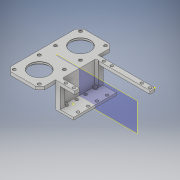
# Autodesk Inventor part: x_carriage_to_extruder
Saved by Autodesk Inventor 2019 (Build 230136000, 136)
## iProperties
Created: 2020-04-12
Part Number: x_carriage_to_extruder
Material: Generisch
Document SubType Name: Modeling
Designer: marc
Density: 1 g/cm^3
Appearance: Vorgabe
Author: marc
Autodesk Inventor part; units mm, degrees
ref_plane "YZ Plane" through (0, 0, 0) normal (1, 0, 0) x (0, 1, 0)
ref_plane "XZ Plane" through (0, 0, 0) normal (0, 1, 0) x (-1, 0, 0)
ref_plane "XY Plane" through (0, 0, 0) normal (0, 0, 1) x (1, 0, 0)
sketch "Skizze1" plane through (0, 0, 0) normal (0, 1, 0) x (-1, 0, 0)
  line L0 (0, 0) -> (70, 0)
  line L1 (70, 0) -> (70, 53)
  line L2 (0, 6) -> (0, 0)
  line L3 (70, 53) -> (0, 53)
  line L4 (0, 53) -> (0, 47)
  line L5 (0, 47) -> (64, 47)
  line L6 (64, 47) -> (64, 6)
  line L7 (64, 6) -> (0, 6)
  dimension "d4" = 53
  dimension "d5" = 6
  dimension "d6" = 6
  dimension "d7" = 70
  dimension "d8" = 6
  constraints: 16 end point, 4 perpendicular, 2 horizontal, 1 parallel, 1 vertical, 1 vertical alignment
  measures "d4" distance between parallel lines of L0 L3
  measures "d5" distance of L2.start L0.start
  measures "d6" distance between parallel lines of L1 L6
  measures "d7" distance of L0.start L0.end
  measures "d8" distance of L3.end L4.end
extrude "Extrusion1" add sketch "Skizze1" along normal blind 4
sketch "Skizze2" plane through (0, 4, 0) normal (0, 1, 0) x (1, 0, 0)
  point P0 (0, 0)
sketch "Skizze3" plane through (-70, 0, 53) normal (0, 0, 1) x (1, 0, 0)
  line L0 (70, 0) -> (0, 0) projected
  line L1 (25, 0) -> (50, 0)
  line L2 (50, 0) -> (50, 1.8)
  line L3 (50, 1.8) -> (25, 1.8)
  line L4 (25, 1.8) -> (25, 0)
  line L5 (70, 0) -> (70, 4) projected
  dimension "d11" = 1.8
  dimension "d12" = 25
  dimension "d13" = 20
  constraints: 8 end point, 2 parallel, 1 horizontal, 1 perpendicular, 1 point on line
  measures "d11" distance of L1.end L2.end
  measures "d12" distance of L2.end L3.end
  measures "d13" distance between parallel lines of L5 L2
extrude "Extrusion2" cut sketch "Skizze3" against normal up to surface (6 mm away)
sketch "Skizze4" plane through (0, 4, 0) normal (0, 1, 0) x (1, 0, 0)
  line L0 (0, -53) -> (0, -47) projected
  line L1 (-70, -53) -> (0, -53) projected
  line L2 (-64, -6) -> (0, -6) projected
  point P0 (0, 0)
  point P1 (-3, -50)
  point P2 (-3, -3)
  point P3 (-60, -50)
  point P4 (-60, -3)
  point P5 (-50, -3)
  point P6 (-50, -50)
  point P7 (-13, -50)
  point P8 (-13, -3)
  dimension "d20" = 3
  dimension "d21" = 3
  dimension "d22" = 6
  dimension "d23" = 3
  dimension "d24" = 10
  dimension "d25" = 37
  dimension "d26" = 10
  constraints: 6 horizontal alignment, 4 vertical alignment
  measures "d20" distance from line of L0 point (-3, -50)
  measures "d21" distance from line of L1 point (-3, -50)
  measures "d22" distance of L0.start L0.end
  measures "d23" distance from line of L2 point (-3, -3)
  measures "d24" distance of point (-3, -50) point (-13, -50)
  measures "d25" distance of point (-50, -50) point (-13, -50)
  measures "d26" distance of point (-50, -50) point (-60, -50)
hole "Bohrung1" at (-60, 4, 50) at (-50, 4, 50) at (-13, 4, 50) at (-3, 4, 50) at (-3, 4, 3) at (-13, 4, 3) at (-50, 4, 3) at (-60, 4, 3) direction (0, -1, 0) diameter 3.6 end through all clearance for "Flachkopfsenkschraube DIN EN ISO 2009" size "M3" standard "DIN"
chamfer "Fase2" distance 1 angle 45 2 edges at (0, 4, 50) (0, 4, 3)
sketch "Skizze6" plane through (0, 0, 0) normal (0, -1, 0) x (1, 0, 0)
  line L0 (-64, 6) -> (-1, 6) projected
  line L1 (-64, 6) -> (-64, 0)
  line L2 (-1, 0) -> (-70, 0) projected
  line L3 (-1, 47) -> (-64, 47) projected
  line L4 (-64, 47) -> (-64, 53)
  line L5 (-70, 53) -> (-1, 53) projected
  line L6 (-64, 47) -> (-64, 6) projected
  line L7 (-70, 0) -> (-70, 53) projected
  point P0 (0, 0)
  constraints: 4 end point, 3 point on line, 1 vertical
extrude "Extrusion3" add sketch "Skizze6" along normal blind 25
sketch "Skizze8" plane through (0, -25, 0) normal (0, -1, 0) x (1, 0, 0)
  line L0 (-70, 0) -> (-70, 53) projected
  line L1 (-70, 53) -> (-54, 53)
  line L2 (-54, 53) -> (-54, 0)
  line L3 (-54, 0) -> (-70, 0)
  line L4 (-70, 0) -> (-70, 53)
  point P0 (0, 0)
  dimension "d40" = 16
  constraints: 8 end point, 2 parallel, 1 horizontal, 1 perpendicular, 1 point on line
  measures "d40" distance of L2.end L3.end
extrude "Extrusion4" add sketch "Skizze8" along normal blind 3
move faces "Verschieben1" translate (6.5, 0, 0) faces at (-54, -27, 17.6667)
sketch "Skizze9" plane through (0, -28, 0) normal (0, -1, 0) x (1, 0, 0)
  line L0 (-70, 53) -> (-70, 0) projected
  line L1 (-47.5, 53) -> (-70, 53) projected
  point P0 (0, 0)
  point P1 (-64.6, 8.5)
  point P2 (-64.6, 21)
  point P3 (-64.6, 32)
  point P4 (-64.6, 44.5)
  point P5 (-50.6, 21)
  point P6 (-50.6, 8.5)
  point P7 (-50.6, 32)
  point P8 (-50.6, 44.5)
  dimension "d43" = 5.4
  dimension "d44" = 12.5
  dimension "d45" = 14
  dimension "d49" = 12.5
  dimension "d50" = 11
  dimension "d51" = 53
  dimension "d52" = 36
  dimension "d53" = 8.5
  constraints: 6 vertical alignment, 4 horizontal alignment
  measures "d43" distance from line of L0 point (-64.6, 21)
  measures "d44" distance of point (-64.6, 8.5) point (-64.6, 21)
  measures "d45" distance of point (-50.6, 21) point (-64.6, 21)
  measures "d49" distance of point (-64.6, 44.5) point (-64.6, 32)
  measures "d50" distance of point (-64.6, 21) point (-64.6, 32)
  measures "d51" distance of L0.start L0.end
  measures "d52" distance of point (-64.6, 8.5) point (-64.6, 44.5)
  measures "d53" distance from line of L1 point (-64.6, 44.5)
hole "Bohrung2" at (-50.6, -28, 8.5) at (-50.6, -28, 21) at (-64.6, -28, 8.5) at (-64.6, -28, 21) at (-50.6, -28, 32) at (-50.6, -28, 44.5) at (-64.6, -28, 44.5) at (-64.6, -28, 32) direction (0, 1, 0) diameter 3.6 end through all clearance for "Flachkopfsenkschraube DIN EN ISO 2009" size "M3" standard "DIN"
sketch "Skizze11" plane through (0, 4, 0) normal (0, 1, 0) x (1, 0, 0)
  arc A0 (-64, -42.8029) -> (-64, -46.1971) centre (-64.6, -44.5) ccw projected
  arc A1 (-64, -19.3029) -> (-64, -22.6971) centre (-64.6, -21) ccw projected
  arc A2 (-64, -6.8029) -> (-64, -10.1971) centre (-64.6, -8.5) ccw projected
  line L0 (-67.45, -42.8546) -> (-64.6, -41.2091)
  line L1 (-64.6, -41.2091) -> (-61.75, -42.8546)
  line L2 (-61.75, -42.8546) -> (-61.75, -46.1454)
  line L3 (-61.75, -46.1454) -> (-64.6, -47.7909)
  line L4 (-64.6, -47.7909) -> (-67.45, -46.1454)
  line L5 (-67.45, -46.1454) -> (-67.45, -42.8546)
  line L6 (-64.6, -11.7909) -> (-67.45, -10.1454)
  line L7 (-67.45, -10.1454) -> (-67.45, -6.8546)
  line L8 (-67.45, -6.8546) -> (-64.6, -5.2091)
  line L9 (-64.6, -5.2091) -> (-61.75, -6.8546)
  line L10 (-61.75, -6.8546) -> (-61.75, -10.1454)
  line L11 (-61.75, -10.1454) -> (-64.6, -11.7909)
  line L12 (-64, -42.8029) -> (-64, -22.6971) projected
  line L13 (-64.6, -24.2909) -> (-67.45, -22.6454)
  line L14 (-67.45, -22.6454) -> (-67.45, -19.3546)
  line L15 (-67.45, -19.3546) -> (-64.6, -17.7091)
  line L16 (-64.6, -17.7091) -> (-61.75, -19.3546)
  line L17 (-61.75, -19.3546) -> (-61.75, -22.6454)
  line L18 (-61.75, -22.6454) -> (-64.6, -24.2909)
  line L19 (-47.5, 0) -> (-47.5, -53) projected
  arc A3 (-64, -30.3029) -> (-64, -33.6971) centre (-64.6, -32) ccw projected
  line L20 (-64.6, -35.2909) -> (-67.45, -33.6454)
  line L21 (-67.45, -33.6454) -> (-67.45, -30.3546)
  line L22 (-67.45, -30.3546) -> (-64.6, -28.7091)
  line L23 (-64.6, -28.7091) -> (-61.75, -30.3546)
  line L24 (-61.75, -30.3546) -> (-61.75, -33.6454)
  line L25 (-61.75, -33.6454) -> (-64.6, -35.2909)
  point P0 (0, 0)
  dimension "d62" = 5.7
  dimension "d64" = 5.7
  constraints: 48 end point, 6 coincident, 4 vertical alignment, 2 parallel, 52 other
  measures "d62" distance between parallel lines of L3 L0
  measures "d64" distance between parallel lines of L24 L21
extrude "Extrusion5" cut sketch "Skizze11" against normal blind 27 contours L0 L1 L2 L3 L4 L5 | L6 L7 L8 L9 L10 L11 | L12 L23 L24 L25 | L12 L25 L20 L21 L22 L23 A3 | L13 L14 L15 L16 L17 L18
sketch "Skizze12" plane through (0, 4, 0) normal (0, 1, 0) x (1, 0, 0)
  line L0 (-61.75, -6.8546) -> (-61.75, -10.1454) projected
  line L1 (-67.45, -42.8546) -> (-64.6, -41.2091) projected
  line L2 (-61.75, -10.1454) -> (-67.45, -10.1454)
  line L3 (-67.45, -10.1454) -> (-67.45, -42.8546)
  line L4 (-67.45, -42.8546) -> (-61.75, -42.8546)
  line L5 (-61.75, -42.8546) -> (-61.75, -10.1454)
  point P0 (0, 0)
  constraints: 8 end point, 2 parallel, 1 horizontal, 1 perpendicular
extrude "Extrusion6" cut sketch "Skizze12" against normal up to surface (29 mm away)
chamfer "Fase3" distance 1.7 angle 45 2 edges at (-20, 1.8, 50) (-45, 1.8, 50)
fillet "Rundung1" radius 2 2 edges at (-20, 0, 50) (-45, 0, 50)
chamfer "Fase4" [suppressed]
sketch "Skizze13" plane through (-64.6, -23, 47.7909) normal (0.5, 0, -0.8660254) x (-0.8660254, 0, -0.5)
  point P0 (-32.0498, 23)
sketch "Skizze15" plane through (0, 0, 0) normal (0, 0, -1) x (-1, 0, 0)
  line L0 (68.3, -28) -> (70, -26.3) projected
  line L1 (70, -26.3) -> (91.2132, -5.0868)
  line L2 (70, -26.3) -> (100, -26.3) construction
  line L3 (91.2132, -5.0868) -> (88.3848, -2.2584)
  line L4 (88.3848, -2.2584) -> (70, -20.6431)
  line L5 (70, -28) -> (70, 4) projected
  point P0 (0, 0)
  point P1 (70, 2.3)
  dimension "d80" = 30
  dimension "d81" = 45
  dimension "d82" = 4
  constraints: 8 end point, 2 perpendicular, 1 collinear, 1 equal length, 1 horizontal, 1 point on line
  measures "d80" distance of L0.end L1.end
  measures "d81" angle of L2 L1
  measures "d82" distance of L1.end L3.end
extrude "Extrusion8" [suppressed]
sketch "Skizze16" plane through (-68.3, -28, 53) normal (-0.7071068, -0.7071068, 0) x (-0.7071068, 0.7071068, 0)
  line L0 (0, 0) -> (2.4042, 0) projected
  line L1 (32.4042, 53) -> (32.4042, 0) projected
  point P0 (-28.4964, 53)
  point P1 (27.0042, 8.5)
  point P2 (13.0042, 8.5)
  point P3 (27.0042, 21)
  point P4 (13.0042, 21)
  point P5 (27.0042, 32)
  point P6 (13.0042, 32)
  point P7 (27.0042, 44.5)
  point P8 (13.0042, 44.5)
  dimension "d85" = 8.5
  dimension "d86" = 36
  dimension "d87" = 11
  dimension "d88" = 12.5
  dimension "d89" = 14
  dimension "d90" = 5.4
  constraints: 6 vertical alignment, 4 horizontal alignment
  measures "d85" distance from line of L0 point (27.004, 8.5)
  measures "d86" distance of point (27.004, 44.5) point (27.004, 8.5)
  measures "d87" distance of point (27.004, 32) point (27.004, 21)
  measures "d88" distance of point (27.004, 44.5) point (27.004, 32)
  measures "d89" distance of point (27.004, 21) point (13.004, 21)
  measures "d90" distance from line of L1 point (27.004, 21)
hole "Bohrung3" [suppressed]
sketch "Skizze17" plane through (0, 0, 53) normal (0, 0, 1) x (1, 0, 0)
  line L0 (-46.2285, 0) -> (0, 0)
  line L1 (0, 0) -> (0, 4)
  line L2 (0, 4) -> (-46.2285, 4)
  line L3 (-46.2285, 4) -> (-46.2285, 0)
  line L4 (-64, 0) -> (-45.6245, 0) projected
  point P0 (0, 0)
  point P1 (-1, 4)
  dimension "d98" = 46.2285
  constraints: 8 end point, 4 point on line, 2 parallel, 1 horizontal, 1 perpendicular
  measures "d98" distance of L1.end L2.end
extrude "Extrusion9" cut sketch "Skizze17" against normal up to surface (6 mm away)
fillet "Rundung2" [suppressed]
sketch "Skizze18" plane through (0, 0, 0) normal (0, 0, -1) x (-1, 0, 0)
  line L0 (70, -28) -> (70, 4) projected
  line L1 (70, -7.7) -> (94.7487, -32.4487)
  line L2 (70, 2.3) -> (105, 2.3) construction
  line L3 (94.7487, -32.4487) -> (91.9203, -35.2772)
  line L4 (91.9203, -35.2772) -> (70, -13.3569)
  line L5 (70, -28) -> (70, 4) projected
  point P0 (0, 0)
  point P1 (70, -26.3)
  dimension "d102" = 35
  dimension "d103" = 45
  dimension "d104" = 4
  dimension "d126" = 10
  constraints: 8 end point, 2 perpendicular, 2 point on line, 1 equal length, 1 horizontal
  measures "d102" distance of L1.start L1.end
  measures "d103" angle of L1 L2
  measures "d104" distance of L1.end L3.end
  measures "d126" distance of L2.start L1.start
extrude "Extrusion10" [suppressed]
sketch "Skizze19" plane through (-68.3, 4, 0) normal (-0.7071068, 0.7071068, 0) x (-0.7071068, -0.7071068, 0)
  line L0 (2.4042, 53) -> (0, 53) projected
  line L1 (0, 53) -> (0, 0) projected
  line L2 (9.4752, 0) -> (9.4752, 53) projected
  point P0 (-45.467, 0)
  point P1 (40.4752, 44.5)
  point P2 (40.4752, 32)
  point P3 (26.4752, 44.5)
  point P4 (26.4752, 32)
  point P5 (26.4752, 21)
  point P6 (26.4752, 8.5)
  point P7 (40.4752, 21)
  point P8 (40.4752, 8.5)
  point P9 (32.4042, 53)
  dimension "d107" = 8.5
  dimension "d108" = 36
  dimension "d109" = 12.5
  dimension "d110" = 11
  dimension "d112" = 14
  dimension "d128" = 17
  constraints: 6 vertical alignment, 4 horizontal alignment
  measures "d107" distance from line of L0 point (40.475, 44.5)
  measures "d108" distance of point (26.475, 8.5) point (26.475, 44.5)
  measures "d109" distance of point (26.475, 44.5) point (26.475, 32)
  measures "d110" distance of point (26.475, 32) point (26.475, 21)
  measures "d112" distance of point (40.475, 32) point (26.475, 32)
  measures "d128" distance from line of L2 point (26.475, 44.5)
hole "Bohrung4" [suppressed]
sketch "Skizze20" plane through (0, 0, 0) normal (0, 0, -1) x (-1, 0, 0)
  line L0 (70, -13.3569) -> (91.9203, -35.2772) projected
  line L1 (76.4716, -19.8284) -> (70, -19.8284)
  line L2 (70, -28) -> (70, 4) projected
  point P0 (0, 0)
  point P1 (70, -26.3)
  point P2 (70, 2.3)
  dimension "d120" = 90
  constraints: 2 end point, 2 point on line
  measures "d120" angle of L2 L1
extrude "Extrusion11" [suppressed]
ref_plane "Arbeitsebene1" through (0, 0, 26.5) normal (0, 0, -1) x (-1, 0, 0)
mirror "Spiegeln1" [suppressed]
pattern_linear "Rechteckige Anordnung1" [suppressed]
sketch "Skizze21" plane through (-70, 4, 0) normal (-1, 0, 0) x (0, 0, 1)
  line L0 (53, -32) -> (53, 0) projected
  line L1 (0, 0) -> (53, 0)
  line L2 (53, 0) -> (53, -4)
  line L3 (53, -4) -> (0, -4)
  line L4 (0, -4) -> (0, 0)
  point P0 (0, -4)
  dimension "d129" = 4
  constraints: 8 end point, 2 parallel, 1 coincident, 1 horizontal, 1 perpendicular, 1 point on line
  measures "d129" distance of L0.end L2.end
extrude "Extrusion12" add sketch "Skizze21" along normal blind 42
sketch "Skizze22" plane through (0, 4, 0) normal (0, 1, 0) x (1, 0, 0)
  line L0 (-134.4, -26.5) -> (22.4, -26.5) projected
  line L1 (-70, -53) -> (-70, 0) projected
  line L2 (-70, -53) -> (-70, 0) projected
  line L3 (-1, 0) -> (-112, 0) projected
  point P0 (0, 0)
  point P1 (-106.5, -16.5)
  point P2 (-75.5, -16.5)
  point P3 (-106.5, 14.5)
  point P4 (-75.5, 14.5)
  dimension "d132" = 10
  dimension "d133" = 31
  dimension "d134" = 5.5
  dimension "d135" = 16.5
  dimension "d138" = 31
  dimension "d139" = 31
  constraints: 2 horizontal alignment, 1 vertical alignment
  measures "d132" distance from line of L0 point (-106.5, -16.5)
  measures "d133" distance of point (-106.5, -16.5) point (-75.5, -16.5)
  measures "d134" distance from line of L1 point (-75.5, -16.5)
  measures "d135" distance from line of L3 point (-75.5, -16.5)
  measures "d138" distance of point (-106.5, -16.5) point (-106.5, 14.5)
  measures "d139" distance of point (-75.5, -16.5) point (-75.5, 14.5)
sketch "Skizze23" plane through (0, 0, 0) normal (0, 0, -1) x (-1, 0, 0)
  line L0 (1, 4) -> (112, 4) projected
  line L1 (112, 0) -> (70, 0)
  line L2 (70, 0) -> (70, 4)
  line L3 (70, 4) -> (112, 4)
  line L4 (112, 4) -> (112, 0)
  point P0 (0, 0)
  point P1 (75.5, 4)
  point P2 (106.5, 4)
  constraints: 8 end point, 2 parallel, 2 point on line, 1 coincident, 1 horizontal, 1 perpendicular
extrude "Extrusion13" add sketch "Skizze23" along normal blind 25.5
hole "Bohrung5" at (-106.5, 4, -14.5) at (-106.5, 4, 16.5) at (-75.5, 4, 16.5) at (-75.5, 4, -14.5) direction (0, -1, 0) diameter 3.4 end through all
sketch "Skizze24" plane through (0, 4, 0) normal (0, 1, 0) x (1, 0, 0)
  circle A0 centre (-106.5, -16.5) radius 1.7 projected
  point P0 (0, 0)
  point P1 (-91, -1)
  dimension "d147" = 15.5
  dimension "d148" = 15.5
  measures "d147" horizontal distance of A0.centre point (-91, -1)
  measures "d148" horizontal distance of A0.centre point (-91, -1)
hole "Bohrung6" at (-91, 4, 1) direction (0, -1, 0) diameter 24 end through all
chamfer "Fase5" distance 2 angle 45 1 edges at (-91, 0, -11)
move faces "Verschieben2" translate (0, 0, 6.5) faces at (-98, 1.3333, -25.5)
chamfer "Fase6" distance 5.25 angle 45 2 edges at (-70, 2, -19) (-112, 2, -19)
mirror "Spiegeln3" about plane through (0, 0, 26.5) normal (0, 0, -1) of "Extrusion13", "Bohrung5", "Bohrung6", "Fase5"
move faces "Verschieben3" translate (0, 0, -6.5) faces at (-98, 1.3333, 78.5)
chamfer "Fase7" distance 5.25 angle 45 2 edges at (-70, 2, 72) (-112, 2, 72)
sketch "Skizze26" plane through (0, 0, 26.5) normal (0, 0, -1) x (-1, 0, 0)
  line L0 (70, 0) -> (90, 0)
  line L1 (90, 0) -> (90, -28)
  line L2 (90, -28) -> (70, -28)
  line L3 (70, -28) -> (70, 0)
  point P0 (0, 0)
  dimension "d173" = 20
  constraints: 8 end point, 2 parallel, 1 horizontal, 1 horizontal alignment, 1 perpendicular
  measures "d173" distance of L2.end L1.end
extrude "Extrusion14" add sketch "Skizze26" along normal blind 0.5
chamfer "Fase8" distance 21 angle 45 1 edges at (-90, -28, 26.25)
chamfer "Fase9" distance 0.2 angle 45 18 edges at (-75.5, 0, -16.2) (-75.5, 0, 14.8) (-106.5, 0, 14.8) (-106.5, 0, -16.2) (-106.5, 0, 38.2) (-75.5, 0, 38.2) (-75.5, 0, 69.2) (-106.5, 4, 69.2) (-106.5, 0, 69.2) (-75.5, 4, -16.2) (-106.5, 4, -16.2) (-75.5, 4, 14.8) (-106.5, 4, 14.8) (-106.5, 4, 38.2) (-75.5, 4, 38.2) (-75.5, 4, 69.2) (-91, 4, 64) (-91, 4, -11)
fillet "Rundung3" radius 0.5 2 edges at (-70, 0, 13) (-70, 0, 39.75)
equation "\"d6\" = d5"
equation "\"d21\" = 0.5 * d22"
equation "\"d23\" = d21"
equation "\"d49\" = d44"
equation "\"d53\" = -0.5 * d52 + 0.5 * d51"
equation "\"d64\" = d62"
equation "\"d147\" = d148"
